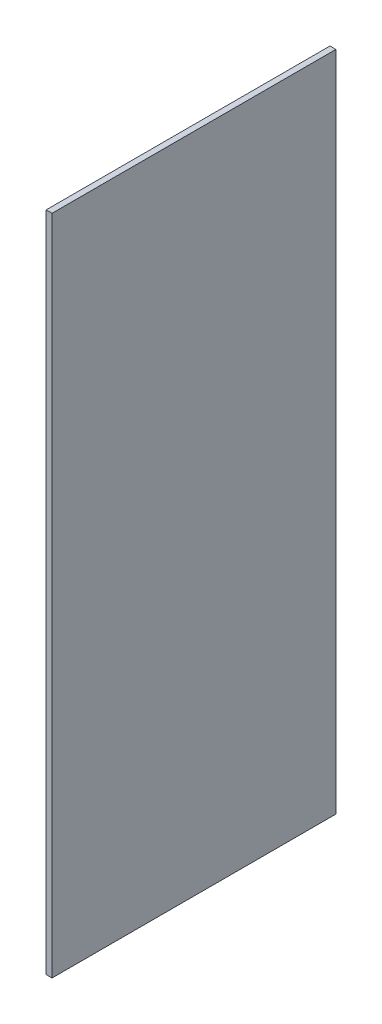
# Autodesk Inventor part: acrylglas
Saved by Autodesk Inventor 2023 (Build 270158000, 158)
## iProperties
Created: 2026-03-17
Part Number: acrylglas
Material: Glas
Document SubType Name: Modeling
Designer: lerat
Density: 2.18 g/cm^3
Appearance: Klar
Author: lerat
Autodesk Inventor part; units mm, degrees
ref_plane "YZ Plane" through (0, 0, 0) normal (1, 0, 0) x (0, 1, 0)
ref_plane "XZ Plane" through (0, 0, 0) normal (0, 1, 0) x (-1, 0, 0)
ref_plane "XY Plane" through (0, 0, 0) normal (0, 0, 1) x (1, 0, 0)
sketch "Skizze1" plane through (0, 0, 0) normal (1, 0, 0) x (0, 1, 0)
  line L0 (112, -48) -> (-112, -48)
  line L1 (-112, -48) -> (-112, 48)
  line L2 (-112, 48) -> (112, 48)
  line L3 (112, 48) -> (112, -48)
  line L4 (112, -48) -> (-112, 48) construction
  line L5 (-112, -48) -> (112, 48) construction
  point P0 (0, 0)
  dimension "d0" = 224
  dimension "d1" = 96
  constraints: 12 end point, 2 midpoint, 2 parallel, 1 horizontal, 1 perpendicular
  measures "d0" distance of L1.end L2.end
  measures "d1" distance of L0.end L1.end
extrude "Extrusion1" add sketch "Skizze1" along normal blind 2
